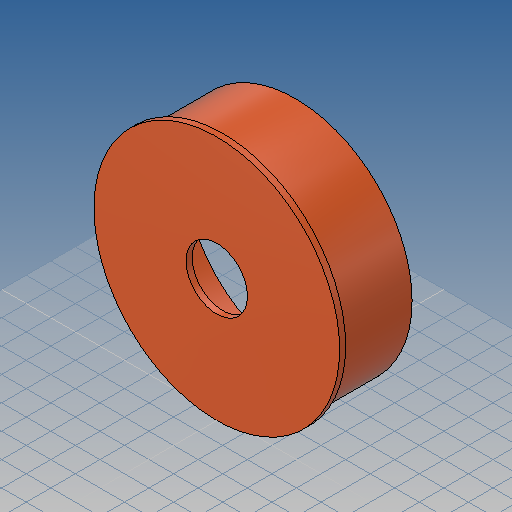
# Autodesk Inventor part: Zyklon_Deckel
Saved by Autodesk Inventor 2019 (Build 230136000, 136)
## iProperties
Created: 2020-07-31
Part Number: Zyklon_Deckel
Material: Generisch
Document SubType Name: Modeling
Designer: Stefan
Mass: 332.609 g
Surface Area: 1312.23 cm^2
Volume: 332.609 cm^3
Density: 1 g/cm^3
Appearance: Glatt - Hellorange
Author: Stefan
Autodesk Inventor part; units mm, degrees
ref_plane "YZ Plane" through (0, 0, 0) normal (1, 0, 0) x (0, 1, 0)
ref_plane "XZ Plane" through (0, 0, 0) normal (0, 1, 0) x (-1, 0, 0)
ref_plane "XY Plane" through (0, 0, 0) normal (0, 0, 1) x (1, 0, 0)
sketch "Skizze1" plane through (0, 0, 0) normal (0, 0, 1) x (1, 0, 0)
  circle A0 centre (0, 0) radius 100
  circle A1 centre (0, 0) radius 95.1
  circle A2 centre (0, 0) radius 89.6
  circle A3 centre (0, 0) radius 25
  dimension "d0" = 200
  dimension "d1" = 4.9
  dimension "d2" = 5.5
  dimension "d7" = 50
  constraints: 4 centre point, 4 coincident
  measures "d0" diameter of A0
  measures "d1" radial gap between concentric circles of A1 A0
  measures "d2" radial gap between concentric circles of A1 A2
  measures "d7" diameter of A3
extrude "Extrusion1" add sketch "Skizze1" along normal blind 4.9 contours A0 | A1 | A2
extrude "Extrusion2" add sketch "Skizze1" against normal blind 59 contours A1
equation "\"d0\" = kg_diameter"
equation "\"d1\" = kg_thickness"
equation "\"d7\" = ht_diameter"
equation "\"d3\" = kg_thickness"
equation "\"kg_diameter\" = 200"
equation "\"kg_thickness\" = 4.9"
equation "\"ht_diameter\" = 50"
equation "\"ht_thickness\" = 1.9"
equation "\"case_thickness\" = 18"
equation "\"gap_fit\" = 0.1"
equation "\"gap_slide\" = 0.2"
equation "\"gap_air\" = 1"
equation "\"bore_diameter\" = 73"
equation "\"tape_thickness\" = 3"
equation "\"mdf_thickness\" = 6"
equation "\"tape_width\" = 15"
equation "\"inner_thickness\" = 15"
equation "\"inner_depth\" = 255"
